Autodesk Inventor part; units mm, degrees
(part 2 of 2)
chamfer "Zkosení5" distance 0.4 angle 70 1 edges at (0, 4.075, 0) measured on face at (0, 4.575, 0)
equation "\"d7\" = d6"
equation "\"d16\" = d15"
equation "\"d17\" = d15"
equation "\"d42\" = d41"
equation "\"d43\" = 0.5 * d41"
equation "\"d44\" = 0.5 * d41"
equation "\"d86\" = d84"
equation "\"d87\" = d84"
equation "\"d89\" = d84"
equation "\"d90\" = d84"
equation "\"d91\" = d84"
equation "\"d92\" = d84"
equation "\"d93\" = d84"
equation "\"d94\" = d84"
equation "\"d98\" = d97"
equation "\"d100\" = d99"
equation "\"d101\" = d99"
equation "\"d104\" = d102"
equation "\"d105\" = d99"
equation "\"d106\" = d99"
equation "\"d107\" = d99"
equation "\"d108\" = d99"
equation "\"d109\" = d99"
equation "\"d113\" = d99"
equation "\"d114\" = d112"
equation "\"d116\" = d115"
equation "\"d117\" = d115"
equation "\"d120\" = d112"
equation "\"d125\" = d99"
equation "\"d95\" = d19 + 2 * d71"
equation "\"rev_num\" = 4"
equation "\"d19\" = 11.95"
equation "\"d71\" = -1"
